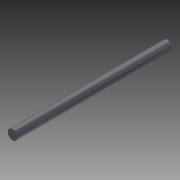
# Autodesk Inventor part: Shooter Conveyor Shaft 0.25 inch
Saved by Autodesk Inventor 2014 SP1 (Build 180222100, 222)
## iProperties
Created: 2012-03-04
Part Number: Shooter Conveyor Shaft 0.25 inch
Material: Steel
Document SubType Name: Modeling
Designer: Moses
Mass: 25.2581 g
Surface Area: 20.9017 cm^2
Volume: 3.21759 cm^3
Density: 7.85 g/cm^3
Appearance: Steel - Polished
Author: Moses
Autodesk Inventor part; units mm, degrees
ref_plane "YZ Plane" through (0, 0, 0) normal (1, 0, 0) x (0, 1, 0)
ref_plane "XZ Plane" through (0, 0, 0) normal (0, 1, 0) x (-1, 0, 0)
ref_plane "XY Plane" through (0, 0, 0) normal (0, 0, 1) x (1, 0, 0)
sketch "Sketch1" plane through (0, 0, 0) normal (0, 0, 1) x (1, 0, 0)
  circle A0 centre (0, 0) radius 3.175
  dimension "d0" = 6.35
  constraints: 1 centre point, 1 coincident
  measures "d0" diameter of A0
extrude "Extrusion1" add sketch "Sketch1" along normal blind 101.6
body "Solid1"
